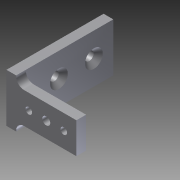
# Autodesk Inventor part: 1_0204_013
Saved by Autodesk Inventor 2012 SP1 (Build 160190100, 190)
## iProperties
Created: 2013-03-28
Part Number: 1_0204_013
Material: Default
Document SubType Name: Modeling
Designer: vogel
Density: 1 g/cm^3
Author: vogel
Autodesk Inventor part; units mm, degrees
ref_plane "YZ Plane" through (0, 0, 0) normal (1, 0, 0) x (0, 1, 0)
ref_plane "XZ Plane" through (0, 0, 0) normal (0, 1, 0) x (-1, 0, 0)
ref_plane "XY Plane" through (0, 0, 0) normal (0, 0, 1) x (1, 0, 0)
sketch "Skizze1" plane through (0, 0, 0) normal (0, 0, 1) x (1, 0, 0)
  line L0 (5, 5) -> (5, 50)
  line L1 (5, 50) -> (0, 50)
  line L2 (0, 50) -> (0, 0)
  line L3 (5, 5) -> (50, 5)
  line L4 (50, 5) -> (50, 0)
  line L5 (-10, 0) -> (60, 0) projected
  line L6 (0, -10) -> (0, 60) projected
  line L7 (0, 0) -> (50, 0)
  dimension "d3" = 5
  dimension "d4" = 5
  dimension "d5" = 50
  dimension "d6" = 50
  constraints: 12 end point, 2 collinear, 2 perpendicular, 1 horizontal, 1 parallel
  measures "d3" distance between parallel lines of L0 L2
  measures "d4" distance between parallel lines of L5 L3
  measures "d5" distance of L1.end L2.end
  measures "d6" distance of L2.end L4.end
extrude "Extrusion1" add sketch "Skizze1" along normal blind 25
sketch "Skizze2" plane through (0, 0, 0) normal (0, -1, 0) x (1, 0, 0)
  line L0 (0, 0) -> (0, 25) projected
  line L1 (50, 0) -> (50, 25) projected
  line L2 (5, 0) -> (5, 25) projected
  line L3 (5, 20.5) -> (36, 20.5)
  line L4 (36, 20.5) -> (36, 4.5)
  line L5 (36, 4.5) -> (5, 4.5)
  line L6 (0, 12.5) -> (50, 12.5)
  line L7 (5, 25) -> (50, 25)
  line L8 (50, 25) -> (50, 0)
  line L9 (50, 0) -> (5, 0)
  line L10 (5, 0) -> (5, 4.5)
  line L11 (5, 20.5) -> (5, 25)
  dimension "d9" = 16
  dimension "d11" = 36
  constraints: 18 end point, 4 parallel, 2 horizontal, 2 midpoint, 2 perpendicular, 1 collinear, 1 point on line, 1 other
  measures "d9" distance between parallel lines of L5 L3
  measures "d11" distance between parallel lines of L4 L0
extrude "Extrusion2" cut sketch "Skizze2" against normal through all contours L9 L2 L5 L4 L6 L1 | L6 L4 L3 L2 L7 L1
sketch "Skizze3" plane through (0, 0, 0) normal (0, -1, 0) x (1, 0, 0)
  line L0 (5, 4.5) -> (36, 4.5) projected
  line L1 (36, 4.5) -> (36, 20.5) projected
  line L2 (36, 20.5) -> (5, 20.5) projected
  line L3 (0, 0) -> (0, 25) projected
  line L4 (36, 12.5) -> (0, 12.5)
  line L5 (20.5, 20.5) -> (20.5, 4.5)
  point P0 (20.5, 12.5)
  constraints: 5 midpoint, 4 end point
hole "Bohrung1" at (20.5, 0, 12.5) direction (0, 1, 0) diameter 4.1 end through all
sketch "Skizze4" plane through (0, 0, 0) normal (0, -1, 0) x (1, 0, 0)
  line L0 (5, 4.5) -> (36, 4.5) projected
  line L1 (36, 4.5) -> (36, 20.5) projected
  line L2 (36, 20.5) -> (5, 20.5) projected
  line L3 (0, 0) -> (0, 25) projected
  line L4 (20.5, 20.5) -> (20.5, 4.5)
  line L5 (0, 12.5) -> (36, 12.5)
  point P0 (11.5, 12.5)
  point P1 (29.5, 12.5)
  dimension "d21" = 18
  constraints: 4 end point, 4 midpoint, 2 point on line, 1 symmetric about line
  measures "d21" distance of point (29.5, 12.5) point (11.5, 12.5)
hole "Bohrung2" at (11.5, 0, 12.5) at (29.5, 0, 12.5) direction (0, 1, 0) diameter 3.4 end through all
fillet "Rundung1" radius 4 2 edges at (5, 2.5, 20.5) (5, 2.5, 4.5)
sketch "Skizze5" plane through (5, 0, 0) normal (1, 0, 0) x (0, 0, -1)
  line L0 (0, 50) -> (-25, 50) projected
  line L1 (-0.5, 5) -> (-24.5, 5) projected
  line L2 (-12.5, 50) -> (-12.5, 9.3168)
  point P0 (-12.5, 40)
  point P1 (-12.5, 22)
  dimension "d30" = 10
  dimension "d31" = 18
  constraints: 2 end point, 2 point on line, 1 midpoint, 1 perpendicular
  measures "d30" distance of L2.start point (-12.5, 40)
  measures "d31" distance of point (-12.5, 22) point (-12.5, 40)
hole "Bohrung3" at (5, 40, 12.5) at (5, 22, 12.5) direction (-1, 0, 0) diameter 4.5 end through all countersink diameter 9.2 countersink angle 90
